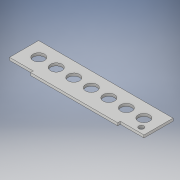
# Autodesk Inventor part: teensy_led_lid
Saved by Autodesk Inventor 2017 (Build 210142000, 142)
## iProperties
Created: 2016-09-21
Part Number: teensy_led_lid
Material: Generic
Document SubType Name: Modeling
Designer: corvera
Density: 1 g/cm^3
Appearance: Default
Author: corvera
Autodesk Inventor part; units mm, degrees
ref_plane "YZ Plane" through (0, 0, 0) normal (1, 0, 0) x (0, 1, 0)
ref_plane "XZ Plane" through (0, 0, 0) normal (0, 1, 0) x (-1, 0, 0)
ref_plane "XY Plane" through (0, 0, 0) normal (0, 0, 1) x (1, 0, 0)
sketch "Sketch1" plane through (0, 0, 0) normal (0, 1, 0) x (-1, 0, 0)
  line L0 (38.35, 8.3) -> (-38.35, 8.3)
  line L1 (-38.35, 8.3) -> (-38.35, -8.3)
  line L2 (-38.35, -8.3) -> (38.35, -8.3)
  line L3 (38.35, -8.3) -> (38.35, 8.3)
  line L4 (38.35, 8.3) -> (-38.35, -8.3) construction
  line L5 (-38.35, 8.3) -> (38.35, -8.3) construction
  line L6 (24.85, 8.3) -> (-24.85, 8.3)
  line L7 (-24.85, 8.3) -> (-24.85, 9.8)
  line L8 (-24.85, 9.8) -> (24.85, 9.8)
  line L9 (24.85, 9.8) -> (24.85, 8.3)
  line L10 (-24.85, 9.8) -> (-38.35, 8.3) construction
  line L11 (24.85, 9.8) -> (38.35, 8.3) construction
  point P0 (0, 0)
  dimension "d0" = 76.7
  dimension "d1" = 16.6
  dimension "d16" = 1.5
  dimension "d17" = 13.5
  constraints: 24 end point, 4 parallel, 2 midpoint, 2 perpendicular, 2 point on line, 1 equal length, 1 horizontal
  measures "d0" distance of L1.end L2.end
  measures "d1" distance of L0.end L1.end
  measures "d16" distance of L6.end L7.end
  measures "d17" distance between parallel lines of L1 L7
extrude "Extrusion1" add sketch "Sketch1" along normal blind 1.5
sketch "Sketch2" plane through (0, 0, 0) normal (0, 1, 0) x (-1, 0, 0)
  circle A0 centre (30, 0) radius 3.25
  line L0 (30, 0) -> (0, 0) construction
  dimension "d4" = 6.5
  dimension "d5" = 30
  constraints: 2 end point, 1 centre point, 1 horizontal
  measures "d4" diameter of A0
  measures "d5" distance of L0.start L0.end
extrude "Extrusion2" cut sketch "Sketch2" along normal through all
pattern_linear "Rectangular Pattern1" count 7 spacing 10 along (1, 0, 0) of "Extrusion2"
sketch "Sketch3" plane through (0, 0, 0) normal (0, 1, 0) x (-1, 0, 0)
  circle A0 centre (-33.85, 5.3) radius 1.45
  line L0 (38.35, -8.3) -> (38.35, 8.3) construction
  line L1 (-33.85, 5.3) -> (-33.85, 8.3) construction
  line L2 (38.35, 8.3) -> (-38.35, 8.3) construction
  line L3 (-33.85, 5.3) -> (-38.35, 5.3) construction
  line L4 (-38.35, 8.3) -> (-38.35, -8.3) construction
  point P0 (0, 0)
  dimension "d11" = 2.9
  dimension "d12" = 3
  dimension "d18" = 4.5
  constraints: 4 end point, 2 point on line, 1 centre point, 1 horizontal, 1 vertical
  measures "d11" diameter of A0
  measures "d12" distance of L1.start L1.end
  measures "d18" distance of L1.start L3.end
extrude "Extrusion3" cut sketch "Sketch3" along normal through all
body "Solid1"
